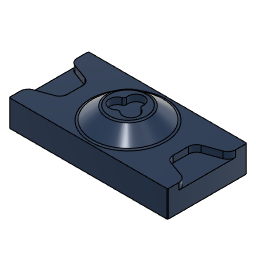
Day #10 v1 (Autodesk Fusion 360 design; units mm, degrees)
Autodesk Fusion 360 part; units mm, degrees
note: some values were not read from the file. Set by a fixed rule: which sketch regions a step uses.
sketch "Sketch1" plane through (0, 0, 0) normal (0, 1, 0) x (1, 0, 0)
  line L0 (76.2, 38.1) -> (-76.2, 38.1)
  line L1 (-76.2, 38.1) -> (-76.2, -38.1)
  line L2 (-76.2, -38.1) -> (76.2, -38.1)
  line L3 (76.2, -38.1) -> (76.2, 38.1)
  line L4 (76.2, 38.1) -> (-76.2, -38.1) construction
  line L5 (-76.2, 38.1) -> (76.2, -38.1) construction
  dimension "d1" = 76.2
  dimension "d2" = 152.4
  constraint perpendicular L0 L1
  constraint parallel L0 L2
  constraint parallel L1 L3
  constraint horizontal L0
  constraint coincident L4 origin
  constraint coincident L5 origin
  measures "d1" distance of L0.end L1.end
  measures "d2" distance of L1.end L2.end
extrude "Extrude1" add sketch "Sketch1" along normal blind 25.4
ref_plane "WorkPlane1" through (0, 38.1, 0) normal (0, 1, 0) x (0, 0, 1)
sketch "Sketch3" plane through (0, 38.1, 0) normal (0, 1, 0) x (1, 0, 0)
  circle A0 centre (0, 0) radius 19.05
  dimension "d6" = 38.1
  constraint coincident A0.centre origin
  measures "d6" diameter of A0
sketch "Sketch4" plane through (0, 25.4, 0) normal (0, 1, 0) x (-1, 0, 0)
  line L0 (-76.2, 38.1) -> (-76.2, -38.1)
  line L1 (-76.2, -38.1) -> (76.2, -38.1)
  line L2 (76.2, -38.1) -> (76.2, 38.1)
  line L3 (76.2, 38.1) -> (-76.2, 38.1)
  circle A0 centre (0, 0) radius 34.925
  dimension "d7" = 69.85
  constraint coincident A0.centre origin
  measures "d7" diameter of A0
loft "Loft1" add profiles "Sketch4", "Sketch3" section 1 contours A0 section 2
fillet "Fillet1" radius 3.175 2 edges at (-17.7608, 38.1, -6.8888) (32.5615, 25.4, 12.6294)
sketch "Sketch5" plane through (0, 25.4, 0) normal (0, 1, 0) x (-1, 0, 0)
  line L0 (-76.2, 38.1) -> (-76.2, -38.1)
  line L1 (-76.2, -38.1) -> (76.2, -38.1)
  line L2 (76.2, -38.1) -> (76.2, 38.1)
  line L3 (76.2, 38.1) -> (-76.2, 38.1)
  circle A0 centre (0, 0) radius 36.0387
  line L4 (76.2, 0) -> (-76.2, 0) construction
  line L5 (-76.2, -21.9448) -> (-50.8, -12.7)
  line L6 (-50.8, -12.7) -> (-50.8, 12.7)
  line L7 (-50.8, 12.7) -> (-76.2, 21.9448)
  line L8 (0, 0) -> (0, -47.7527) construction
  line L9 (50.8, 12.7) -> (76.2, 21.9448)
  line L10 (50.8, -12.7) -> (50.8, 12.7)
  line L11 (76.2, -21.9448) -> (50.8, -12.7)
  dimension "d10" = 25.4
  dimension "d11" = 25.4
  dimension "d12" = 70
  constraint midpoint L2 L4.start
  constraint midpoint L0 L4.end
  constraint coincident L0 L5.start
  constraint perpendicular L4 L6
  constraint coincident L0 L7.end
  constraint symmetric L4 L5.start L7.end
  constraint symmetric L4 L5.end L6.end
  constraint coincident A0.centre L8.start
  constraint perpendicular L1 L8
  constraint symmetric L5.start L8 L11.start
  constraint symmetric L5.end L8 L10.start
  constraint symmetric L6.end L8 L9.start
  constraint symmetric L7.end L8 L9.end
  measures "d10" vertical distance of L5.end L6.end
  measures "d11" distance of L0 L6
  measures "d12" angle of L0 L5
extrude "Extrude2" cut sketch "Sketch5" against normal blind 6.35 contours L0 L5 L6 L7 | L2 L9 L10 L11
fillet "Fillet2" radius 7.62 8 edges at (76.2, 22.225, -21.9448) (76.2, 22.225, 21.9448) (50.8, 22.225, -12.7) (50.8, 22.225, 12.7) (-50.8, 22.225, 12.7) (-50.8, 22.225, -12.7) (-76.2, 22.225, -21.9448) (-76.2, 22.225, 21.9448)
sketch "Sketch6" plane through (0, 38.1, 0) normal (0, 1, 0) x (-1, 0, 0)
  circle A0 centre (0, 0) radius 17.9363
  circle A1 centre (0, -7.62) radius 7.62
  circle A2 centre (6.5991, 3.81) radius 7.62
  circle A3 centre (-6.5991, 3.81) radius 7.62
  dimension "d16" = 15.24
  dimension "d17" = 7.62
  dimension "d19" = 360
  constraint vertical A0.centre A1.centre
  measures "d16" diameter of A1
  measures "d17" vertical distance of A0.centre A1.centre
extrude "Extrude3" cut sketch "Sketch6" against normal blind 6.35 contours A1 A2 A3 | A1 A2 | A1 A2 A3 | A1 A2 A3 | A1 A3 | A2 A3
fillet "Fillet3" radius 2.54 3 edges at (-6.5991, 34.925, -3.81) (6.5991, 34.925, -3.81) (0, 34.925, 7.62)
chamfer "Chamfer2" distance 0.635 angle 45 4 edges at (76.2, 12.7, 38.1) (-76.2, 12.7, 38.1) (-76.2, 12.7, -38.1) (76.2, 12.7, -38.1)
